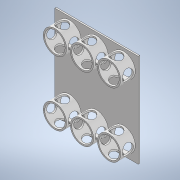
# Autodesk Inventor part: vial holder 2
Saved by Autodesk Inventor 2022 (Build 260153000, 153)
## iProperties
Created: 2022-05-06
Part Number: vial holder 2
Material: Generic
Document SubType Name: Modeling
Designer: efred
Density: 1 g/cm^3
Appearance: Default
Author: efred
Autodesk Inventor part; units mm, degrees
ref_plane "YZ Plane" through (0, 0, 0) normal (1, 0, 0) x (0, 1, 0)
ref_plane "XZ Plane" through (0, 0, 0) normal (0, 1, 0) x (-1, 0, 0)
ref_plane "XY Plane" through (0, 0, 0) normal (0, 0, 1) x (1, 0, 0)
sketch "Sketch1" plane through (0, 0, 0) normal (0, 0, 1) x (1, 0, 0)
  circle A0 centre (41.875, 108.01) radius 13.75 construction
  circle A1 centre (4.875, 108.01) radius 13.75 construction
  circle A2 centre (-32.125, 108.01) radius 13.75 construction
  circle A3 centre (41.875, 20.01) radius 13.75 construction
  circle A4 centre (4.875, 20.01) radius 13.75 construction
  circle A5 centre (-32.125, 20.01) radius 13.75 construction
  line L0 (61.875, 0.01) -> (-52.125, 0.01)
  line L1 (-52.125, 0.01) -> (-52.125, 128.01)
  line L2 (-52.125, 128.01) -> (61.875, 128.01)
  line L3 (61.875, 128.01) -> (61.875, 0.01)
  circle A6 centre (41.875, 20.01) radius 13.95
  circle A7 centre (4.875, 20.01) radius 13.95
  circle A8 centre (-32.125, 20.01) radius 13.95
  circle A9 centre (41.875, 108.01) radius 13.95
  circle A10 centre (4.875, 108.01) radius 13.95
  circle A11 centre (-32.125, 108.01) radius 13.95
  point P0 (0, 0)
  dimension "d0" = 20
  dimension "d1" = 20
  dimension "d2" = 20
  dimension "d3" = 20
  dimension "d4" = 0.2
  dimension "d5" = 0.2
  dimension "d6" = 0.2
  dimension "d7" = 0.2
  dimension "d8" = 0.2
  dimension "d9" = 0.2
  constraints: 8 end point, 6 centre point, 2 parallel, 1 horizontal, 1 perpendicular
  measures "d0" distance from line of A3.centre L3
  measures "d1" distance from line of L0 A3.centre
  measures "d2" distance from line of A5.centre L1
  measures "d3" distance from line of A2.centre L2
  measures "d4" radial gap between concentric circles of A3 A6
  measures "d5" radial gap between concentric circles of A4 A7
  measures "d6" radial gap between concentric circles of A5 A8
  measures "d7" radial gap between concentric circles of A0 A9
  measures "d8" radial gap between concentric circles of A1 A10
  measures "d9" radial gap between concentric circles of A2 A11
extrude "Extrusion1" add sketch "Sketch1" along normal blind 2
sketch "Sketch2" plane through (0, 0, 2) normal (0, 0, 1) x (1, 0, 0)
  line L0 (61.875, 128.01) -> (-52.125, 128.01) projected
  line L1 (-52.125, 128.01) -> (-52.125, 0.01) projected
  line L2 (-52.125, 0.01) -> (61.875, 0.01) projected
  line L3 (61.875, 0.01) -> (61.875, 128.01) projected
  circle A0 centre (-32.125, 108.01) radius 13.95 projected
  circle A1 centre (4.875, 108.01) radius 13.95 projected
  circle A2 centre (41.875, 108.01) radius 13.95 projected
  circle A3 centre (-32.125, 20.01) radius 13.95 projected
  circle A4 centre (4.875, 20.01) radius 13.95 projected
  circle A5 centre (41.875, 20.01) radius 13.95 projected
  circle A6 centre (41.875, 20.01) radius 15.95
  circle A7 centre (4.875, 20.01) radius 15.95
  circle A8 centre (-32.125, 20.01) radius 15.95
  circle A9 centre (41.875, 108.01) radius 15.95
  circle A10 centre (4.875, 108.01) radius 15.95
  circle A11 centre (-32.125, 108.01) radius 15.95
  point P0 (0, 0)
  dimension "d12" = 2
  dimension "d13" = 2
  dimension "d14" = 2
  dimension "d15" = 2
  dimension "d16" = 2
  dimension "d17" = 2
  constraints: 6 centre point
  measures "d12" radial gap between concentric circles of A5 A6
  measures "d13" radial gap between concentric circles of A4 A7
  measures "d14" radial gap between concentric circles of A3 A8
  measures "d15" radial gap between concentric circles of A2 A9
  measures "d16" radial gap between concentric circles of A1 A10
  measures "d17" radial gap between concentric circles of A0 A11
extrude "Extrusion2" add sketch "Sketch2" along normal blind 20 contours A6 | A7 | A8 | A9 | A10 | A11
sketch "Sketch3" plane through (0, 0, 0) normal (1, 0, 0) x (0, 1, 0)
  line L0 (35.96, 22) -> (4.06, 22) projected
  line L1 (4.06, 2) -> (35.96, 2) projected
  line L2 (123.96, 22) -> (92.06, 22) projected
  line L3 (92.06, 2) -> (123.96, 2) projected
  circle A0 centre (20.01, 12) radius 7.5
  circle A1 centre (108.01, 12) radius 7.5
  line L4 (35.96, 2) -> (35.96, 22) projected
  point P0 (0, 0)
  point P1 (35.96, 12)
  point P2 (20.01, 22)
  point P3 (108.01, 22)
  dimension "d20" = 15
  dimension "d21" = 15
  constraints: 3 midpoint, 2 centre point, 2 horizontal alignment, 2 vertical alignment
  measures "d20" diameter of A0
  measures "d21" diameter of A1
extrude "Extrusion3" cut sketch "Sketch3" along normal through all both and the other way through all
sketch "Sketch4" plane through (0, 0, 0) normal (0, 1, 0) x (-1, 0, 0)
  line L0 (48.075, 22) -> (16.175, 22) projected
  line L1 (16.175, 2) -> (48.075, 2) projected
  line L2 (11.075, 22) -> (-20.825, 22) projected
  line L3 (-20.825, 2) -> (11.075, 2) projected
  line L4 (-25.925, 22) -> (-57.825, 22) projected
  line L5 (-57.825, 2) -> (-25.925, 2) projected
  circle A0 centre (32.125, 12) radius 7.5
  circle A1 centre (-4.875, 12) radius 7.5
  circle A2 centre (-41.875, 12) radius 7.5
  point P0 (0, 0)
  point P1 (18.0483, 12)
  point P2 (46.2017, 12)
  point P3 (-18.9517, 12)
  point P4 (9.2017, 12)
  point P5 (-55.9517, 12)
  point P6 (-27.7983, 12)
  point P7 (32.125, 22)
  point P8 (-4.875, 22)
  point P9 (-41.875, 22)
  dimension "d24" = 15
  dimension "d25" = 15
  dimension "d26" = 15
  constraints: 3 centre point, 3 horizontal alignment, 3 midpoint, 3 vertical alignment
  measures "d24" diameter of A0
  measures "d25" diameter of A1
  measures "d26" diameter of A2
extrude "Extrusion4" cut sketch "Sketch4" along normal through all
equation "\"d5\" = d4"
equation "\"d6\" = d4"
equation "\"d7\" = d4"
equation "\"d8\" = d4"
equation "\"d9\" = d4"
equation "\"d20\" = d21"
body "Solid1"
